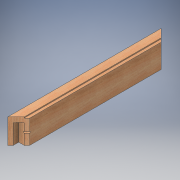
# Autodesk Inventor part: SideLengthOutlet
Saved by Autodesk Inventor 2016 (Build 200138000, 138)
## iProperties
Created: 2016-02-09
Part Number: SideLengthOutlet
Material: Wood (Birch)
Document SubType Name: Modeling
Designer: ron
Density: 0.55 g/cm^3
Appearance: Birch - Natural Polished
Mass: 9097.97 g
Surface Area: 6449.03 cm^2
Volume: 16541.8 cm^3
Author: ron
Autodesk Inventor part; units mm, degrees
ref_plane "YZ Plane" through (0, 0, 0) normal (1, 0, 0) x (0, 1, 0)
ref_plane "XZ Plane" through (0, 0, 0) normal (0, 1, 0) x (-1, 0, 0)
ref_plane "XY Plane" through (0, 0, 0) normal (0, 0, 1) x (1, 0, 0)
sketch "Sketch1" plane through (0, 0, 0) normal (0, 0, 1) x (1, 0, 0)
  line L0 (0, 0) -> (0, 228.6)
  line L1 (0, 228.6) -> (76.2, 228.6)
  line L2 (76.2, 228.6) -> (76.2, 219.2528)
  line L3 (76.2, 219.2528) -> (101.6, 219.2528)
  line L4 (101.6, 219.2528) -> (101.6, 0)
  line L5 (101.6, 0) -> (0, 0)
  dimension "d0" = 228.6
  dimension "d1" = 76.2
  dimension "d2" = 9.3472
  dimension "d3" = 25.4
  constraints: 12 end point, 5 perpendicular, 1 vertical
  measures "d0" distance of L0.start L0.end
  measures "d1" distance of L0.end L1.end
  measures "d2" distance of L1.end L2.end
  measures "d3" distance of L2.end L3.end
extrude "Extrusion1" add sketch "Sketch1" along normal blind 1422.4
ref_plane "Work Plane2" through (25.4038, 0, 736.5962) normal (0, -1, 0) x (1, 0, 0)
sketch "Sketch7" plane through (25.4038, 0, 736.5962) normal (0, -1, 0) x (1, 0, 0)
  line L0 (76.1962, -634.9962) -> (50.7962, -660.3962)
  line L1 (50.7962, -660.3962) -> (-0.0038, -660.3962)
  line L2 (76.1962, -634.9962) -> (-25.4038, -736.5962) projected
  line L3 (76.1962, -736.5962) -> (76.1962, 584.2038) projected
  line L4 (-0.0038, -660.3962) -> (-0.0038, -711.1962)
  line L5 (-0.0038, -711.1962) -> (50.7962, -660.3962)
  dimension "d39" = 50.8
  dimension "d41" = 90
  dimension "d42" = 50.8
  constraints: 8 end point, 1 collinear, 1 point on line
  measures "d39" distance of L0.end L1.end
  measures "d41" angle of L3 L1
  measures "d42" distance of L1.end L4.end
extrude "Extrusion5" cut sketch "Sketch7" against normal blind 181.1528
sketch "Sketch8" plane through (25.4, 0, 76.2) normal (0, -1, 0) x (1, 0, 0)
  line L0 (76.2, -76.2) -> (76.2, 1346.2) projected
  line L1 (76.2, 1244.6) -> (50.8, 1270)
  line L2 (50.8, 1270) -> (0, 1270)
  line L3 (0, 1270) -> (0, 1320.8)
  line L4 (0, 1320.8) -> (50.8, 1270)
  line L5 (-25.4, 1346.2) -> (76.2, 1244.6) projected
  point P0 (-25.4, -76.2)
  point P1 (76.2, 25.4)
  dimension "d48" = 90
  dimension "d49" = 50.8
  constraints: 8 end point, 1 collinear, 1 vertical
  measures "d48" angle of L0 L2
  measures "d49" distance of L1.end L2.end
extrude "Extrusion6" cut sketch "Sketch8" against normal blind 181.1528
chamfer "Chamfer6" distance 101.6 angle 45 1 edges at (101.6, 109.6264, 1422.4)
chamfer "Chamfer7" distance 101.6 angle 45 1 edges at (101.6, 109.6264, 0)
ref_plane "Work Plane4" through (137.521, 56.9702, 1284.879) normal (0.7071068, 0, -0.7071068) x (0, 1, 0)
sketch "Sketch9" plane through (137.521, 56.9702, 1284.879) normal (0.7071068, 0, -0.7071068) x (0, 1, 0)
  line L0 (162.2826, -862.1046) -> (162.2826, 0) projected
  line L1 (162.2826, 0) -> (48.0842, 0)
  line L2 (-56.9702, 0) -> (162.2826, 0) projected
  point P0 (-56.9702, -1005.7887)
  dimension "d63" = 114.1984
  constraints: 2 end point, 1 point on line
  measures "d63" distance of L0.end L1.end
hole "Hole1" at (137.521, 105.0544, 1284.879) direction (-0.7071068, 0, 0.7071068) diameter 12.7 depth 101.6 tip angle 118
sketch "Sketch10" plane through (25.4, 181.1528, 76.2) normal (0, -1, 0) x (1, 0, 0)
  line L0 (50.8, 1270) -> (0, 1270) projected
  line L1 (50.8, 1270) -> (38.1019, 1282.6981)
  line L2 (38.1019, 1282.6981) -> (12.7019, 1282.6981)
  line L3 (12.7019, 1282.6981) -> (12.7019, 1308.0981)
  line L4 (12.7019, 1308.0981) -> (38.1019, 1282.6981)
  point P0 (-25.4, -76.2)
  dimension "d71" = 17.9578
  dimension "d72" = 25.4
  dimension "d73" = 25.4
  constraints: 8 end point, 1 horizontal, 1 perpendicular
  measures "d71" distance of L0.start L1.end
  measures "d72" distance of L1.end L2.end
  measures "d73" distance of L2.end L3.end
extrude "Extrusion7" cut sketch "Sketch10" against normal blind 3.175
sketch "Sketch11" plane through (25.4038, 181.1528, 736.5962) normal (0, -1, 0) x (1, 0, 0)
  line L0 (-0.0038, -660.3962) -> (50.7962, -660.3962) projected
  line L1 (50.7962, -660.3962) -> (38.0981, -673.0942)
  line L2 (38.0981, -673.0942) -> (12.6981, -673.0942)
  line L3 (12.6981, -673.0942) -> (12.6981, -698.4942)
  line L4 (38.0981, -673.0942) -> (12.6981, -698.4942)
  point P0 (-25.4038, -736.5962)
  dimension "d76" = 17.9578
  dimension "d77" = 25.4
  dimension "d78" = 25.4
  constraints: 8 end point, 1 horizontal, 1 perpendicular
  measures "d76" distance of L0.end L1.end
  measures "d77" distance of L1.end L2.end
  measures "d78" distance of L2.end L3.end
extrude "Extrusion8" cut sketch "Sketch11" against normal blind 3.175
body "Solid1"
